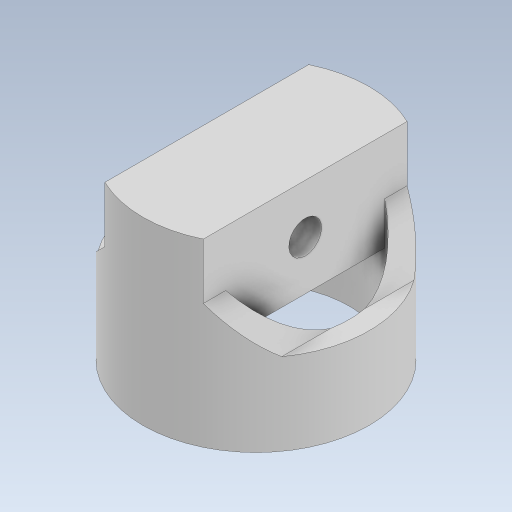
# Autodesk Inventor part: terminal_end_4.1mm_5.7mm_addon_reinforced
Saved by Autodesk Inventor 2024 (Build 280153000, 153)
## iProperties
Created: 2024-04-25
Part Number: terminal_end_4.1mm_5.7mm_addon_reinforced
Material: 일반
Document SubType Name: Modeling
Designer: Gihyeok Na
Density: 1 g/cm^3
Appearance: 기본값
Author: Gihyeok Na
Autodesk Inventor part; units mm, degrees
ref_plane "YZ Plane" through (0, 0, 0) normal (1, 0, 0) x (0, 1, 0)
ref_plane "XZ Plane" through (0, 0, 0) normal (0, 1, 0) x (-1, 0, 0)
ref_plane "XY Plane" through (0, 0, 0) normal (0, 0, 1) x (1, 0, 0)
sketch "스케치1" plane through (0, 0, 0) normal (0, 1, 0) x (-1, 0, 0)
  circle A0 centre (0, 0) radius 2.85
  circle A1 centre (0, 0) radius 3.45
  dimension "d0" = 5.7
  dimension "d1" = 6.9
  constraints: 2 centre point, 2 coincident
  measures "d0" diameter of A0
  measures "d1" diameter of A1
extrude "돌출1" add sketch "스케치1" along normal blind 2.5
sketch "스케치2" plane through (0, 2.5, 0) normal (0, 1, 0) x (1, 0, 0)
  circle A0 centre (0, 0) radius 3.45 projected
  circle A1 centre (0, 0) radius 3.45 projected
  line L0 (1.5, 3.1068) -> (-1.5, 3.1068)
  line L1 (-1.5, 3.1068) -> (-1.5, -3.1068)
  line L2 (-1.5, -3.1068) -> (1.5, -3.1068)
  line L3 (1.5, -3.1068) -> (1.5, 3.1068)
  line L4 (1.5, 3.1068) -> (-1.5, -3.1068) construction
  line L5 (-1.5, 3.1068) -> (1.5, -3.1068) construction
  dimension "d4" = 3
  constraints: 12 end point, 2 midpoint, 2 parallel, 1 horizontal, 1 perpendicular, 1 point on circle
  measures "d4" distance of L2.end L1.end
extrude "돌출2" add sketch "스케치2" along normal blind 3 contours L0 A0 | L3 L2 L1 L0 | A0 L2
chamfer "모따기3" distance 1.3 angle 45 4 edges at (1.5, 2.5, 2.7651) (1.5, 2.5, -2.7651) (-1.5, 2.5, 2.7651) (-1.5, 2.5, -2.7651)
sketch "스케치6" plane through (0, 0, 0) normal (1, 0, 0) x (0, 1, 0)
  circle A0 centre (4, 0) radius 0.5
  line L0 (3.8, -2.4233) -> (3.8, -3.1068) projected
  line L1 (3.8, -2.4233) -> (2.5, -2.4233) projected
  line L2 (2.5, -2.4233) -> (2.5, 2.4233) projected
  line L3 (2.5, 2.4233) -> (3.8, 2.4233) projected
  line L4 (3.8, 3.1068) -> (3.8, 2.4233) projected
  line L5 (3.8, 3.1068) -> (5.5, 3.1068) projected
  line L6 (5.5, -3.1068) -> (5.5, 3.1068) projected
  line L7 (3.8, -3.1068) -> (5.5, -3.1068) projected
  point P0 (0, 0)
  dimension "d22" = 1
  dimension "d23" = 1.5
  constraints: 1 centre point
  measures "d22" diameter of A0
  measures "d23" distance from line of L6 A0.centre
extrude "돌출5" cut sketch "스케치6" along normal mid plane 10 contours A0
